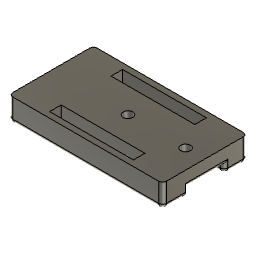
xiao-esp32-bracket v1 (Autodesk Fusion 360 design; units mm, degrees)
Autodesk Fusion 360 part; units mm, degrees
sketch "Sketch1" plane through (0, 0, 0) normal (0, 0, 1) x (1, 0, 0)
  line L0 (10.9, 9.5) -> (-10.9, 9.5)
  line L1 (-10.9, 9.5) -> (-10.9, -9.5)
  line L2 (-10.9, -9.5) -> (10.9, -9.5)
  line L3 (10.9, -9.5) -> (10.9, 9.5)
  line L4 (10.9, 9.5) -> (-10.9, -9.5) construction
  line L5 (-10.9, 9.5) -> (10.9, -9.5) construction
  line L6 (20, -11) -> (-20, -11)
  line L7 (-20, -11) -> (-20, 11)
  line L8 (-20, 11) -> (20, 11)
  line L9 (20, 11) -> (20, -11)
  line L10 (20, -11) -> (-20, 11) construction
  line L11 (-20, -11) -> (20, 11) construction
  line L12 (-10.9, -9.5) -> (10.9, -9.5)
  line L13 (10.9, -9.5) -> (10.9, -6.5)
  line L14 (10.9, -6.5) -> (-10.9, -6.5)
  line L15 (-10.9, -6.5) -> (-10.9, -9.5)
  line L16 (-10.9, 9.5) -> (10.9, 9.5)
  line L17 (10.9, 9.5) -> (10.9, 6.5)
  line L18 (10.9, 6.5) -> (-10.9, 6.5)
  line L19 (-10.9, 6.5) -> (-10.9, 9.5)
  line L20 (20, 5) -> (10, 5)
  line L21 (10, 5) -> (10, -5)
  line L22 (10, -5) -> (20, -5)
  line L23 (20, -5) -> (20, 5)
  line L24 (20, 5) -> (10, -5) construction
  line L25 (10, 5) -> (20, -5) construction
  circle A0 centre (15, 0) radius 1.25
  circle A1 centre (0, 0) radius 1.25
  point P0 (15, 0)
  dimension "d1" = 21.8
  dimension "d2" = 19
  dimension "d3" = 40
  dimension "d4" = 22
  dimension "d9" = 21.8
  dimension "d10" = 3
  dimension "d11" = 21.8
  dimension "d12" = 3
  dimension "d15" = 10
  dimension "d16" = 10
  dimension "d19" = 2.5
  dimension "d20" = 2.5
  constraint horizontal L0
  constraint perpendicular L0 L1
  constraint parallel L0 L2
  constraint parallel L1 L3
  constraint coincident L4 A1.centre
  constraint coincident L5 A1.centre
  constraint coincident A1.centre origin
  constraint horizontal L6
  constraint perpendicular L6 L7
  constraint parallel L6 L8
  constraint parallel L7 L9
  constraint coincident L10 A1.centre
  constraint coincident L11 A1.centre
  constraint horizontal L12
  constraint vertical L13
  constraint horizontal L14
  constraint vertical L15
  constraint horizontal L16
  constraint vertical L17
  constraint horizontal L18
  constraint vertical L19
  constraint horizontal L20
  constraint perpendicular L20 L21
  constraint parallel L20 L22
  constraint parallel L21 L23
  constraint coincident L24 P0
  constraint coincident L25 P0
  constraint coincident P0 A0.centre
  measures "d1" distance of L1.end L2.end
  measures "d2" distance of L0.end L1.end
  measures "d3" distance of L7.end L8.end
  measures "d4" distance of L6.end L7.end
  measures "d9" distance of L1.end L2.end
  measures "d10" distance of L1.end L14.end
  measures "d11" distance of L0.end L0.start
  measures "d12" distance of L0.end L18.end
  measures "d15" distance of L21.end L22.end
  measures "d16" distance of L20.end L21.end
  measures "d19" diameter of A0
  measures "d20" diameter of A1
extrude "Extrude1" add sketch "Sketch1" along normal blind 6 contours L0 L1 L3 L16 L17 L18 L19 | L0 L1 L2 L3 L6 L7 L8 L9 L12 L13 L15 L16 L17 L19 L20 L22 | L1 L3 L14 L18 L20 L21 L22 | L3 L9 L20 L22 L23 | L3 L20 L21 L22 | L1 L2 L3 L12 L13 L14 L15 | A0 | A1
extrude "Extrude2" cut sketch "Sketch1" along normal blind 2 contours L0 L1 L3 L16 L17 L18 L19 | L1 L3 L14 L18 L20 L21 L22 | L3 L20 L21 L22 | L1 L2 L3 L12 L13 L14 L15 | A1
extrude "Extrude3" cut sketch "Sketch1" along normal blind 6 contours L0 L1 L3 L16 L17 L18 L19 | L1 L2 L3 L12 L13 L14 L15
extrude "Extrude4" cut sketch "Sketch1" along normal blind 2 contours L3 L9 L20 L22 L23 | A0
extrude "Extrude5" cut sketch "Sketch1" along normal blind 6 contours A0 | A1
chamfer "Chamfer1" distance 2 angle 45 2 edges at (-1.1654, -0.452, 2) (13.8346, -0.452, 2)
fillet "Fillet1" radius 1 18 edges at (20, 0, 2) (20, 5, 1) (15.45, 5, 0) (10.9, 7.25, 0) (0, 11, 0) (20, 8, 0) (0, -11, 0) (20, -8, 0) (10.9, -7.25, 0) (15.45, -5, 0) (0, -9.5, 0) (-10.9, 0, 0) (0, 9.5, 0) (0, 6.5, 2) (0, -6.5, 2) (-20, 0, 0) (10.9, 5, 1) (10.9, -5, 1)
fillet "Fillet2" radius 1 8 edges at (19.7071, -10.7071, 0.2929) (20, -11, 3.5) (19.7071, 10.7071, 0.2929) (20, 11, 3.5) (-19.7071, -10.7071, 0.2929) (-20, -11, 3.5) (-19.7071, 10.7071, 0.2929) (-20, 11, 3.5)
sketch "Sketch2" plane through (0, 0, 0) normal (0, 0, -1) x (1, 0, 0)
  line L0 (-11.9, -10) -> (-11.9, 10)
  line L1 (-11.9, 10) -> (-19, 10)
  line L2 (-19, 10) -> (-19, -10)
  line L3 (-19, -10) -> (-11.9, -10)
  line L4 (-22, 2) -> (-10, 2)
  line L5 (-10, 2) -> (-10, -2)
  line L6 (-10, -2) -> (-22, -2)
  line L7 (-22, -2) -> (-22, 2)
  line L8 (-22, 2) -> (-10, -2) construction
  line L9 (-10, 2) -> (-22, -2) construction
  point P0 (-16, 0)
  dimension "d28" = 12
  dimension "d29" = 4
  constraint horizontal L4
  constraint perpendicular L4 L5
  constraint parallel L4 L6
  constraint parallel L5 L7
  constraint coincident L8 P0
  constraint coincident L9 P0
  measures "d28" distance of L5.end L6.end
  measures "d29" distance of L4.end L5.end
extrude "Extrude6" cut sketch "Sketch2" against normal blind 2 contours L0 L2 L4 L6 | L0 L4 L5 L6 | L2 L4 L6 L7
fillet "Fillet3" radius 1 10 edges at (-10.9, 2, 1.5) (-11.1929, 2, 0.2929) (-15.45, 2, 0) (-19.7071, 2, 0.2929) (-20, 2, 1.5) (-20, -2, 1.5) (-19.7071, -2, 0.2929) (-15.45, -2, 0) (-11.1929, -2, 0.2929) (-10.9, -2, 1.5)
